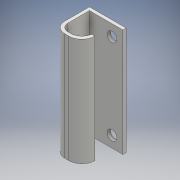
# Autodesk Inventor part: TopHook
Saved by Autodesk Inventor 2016 (Build 200138000, 138)
## iProperties
Created: 2015-06-09
Part Number: TopHook
Material: Generic
Document SubType Name: Modeling
Designer: Erin
Density: 1 g/cm^3
Appearance: Default
Author: Erin
Autodesk Inventor part; units mm, degrees
ref_plane "YZ Plane" through (0, 0, 0) normal (1, 0, 0) x (0, 1, 0)
ref_plane "XZ Plane" through (0, 0, 0) normal (0, 1, 0) x (-1, 0, 0)
ref_plane "XY Plane" through (0, 0, 0) normal (0, 0, 1) x (1, 0, 0)
sketch "Sketch1" plane through (0, 0, 0) normal (0, 0, 1) x (1, 0, 0)
  line L0 (-3.7865, -1.449) -> (13.2135, -1.449)
  line L1 (13.2135, -1.449) -> (13.2135, -2.949)
  line L2 (13.2135, -2.949) -> (-3.7865, -2.949)
  line L3 (-3.7865, -2.949) -> (-3.7865, -1.449)
  line L4 (-3.7865, -2.949) -> (-2.2865, -2.949)
  line L5 (-3.7865, -12.949) -> (-3.7865, -2.949)
  line L6 (3.2135, -16.449) -> (3.2135, -17.949)
  line L7 (3.2135, -17.949) -> (1.2135, -17.949)
  arc A0 (3.2135, -16.449) -> (7.7135, -11.949) centre (2.4495, -11.1849) ccw
  line L8 (7.7135, -11.949) -> (9.2135, -11.949)
  arc A1 (3.2135, -17.949) -> (9.2135, -11.949) centre (3.2135, -11.949) ccw
  arc A2 (-3.7865, -12.949) -> (1.2135, -17.949) centre (1.2135, -12.949) ccw
  arc A3 (-2.2865, -12.949) -> (1.2135, -16.449) centre (1.2135, -12.949) ccw
  line L9 (-3.7865, -12.949) -> (-2.2865, -12.949)
  line L10 (1.2135, -17.949) -> (1.2135, -16.449)
  line L11 (1.2135, -16.449) -> (3.2135, -16.449)
  line L12 (-2.2865, -2.949) -> (-2.2865, -12.949)
  point P0 (0, 0)
  dimension "d0" = 1.5
  dimension "d2" = 1.5
  dimension "d3" = 6
  dimension "d4" = 5
  dimension "d5" = 5
  dimension "d7" = 6
  dimension "d8" = 2
  dimension "d12" = 15.5
  dimension "d13" = 10
  dimension "d23" = 1.5
  constraints: 26 end point, 10 point on circle, 5 horizontal, 4 centre point, 4 parallel, 3 perpendicular, 2 point on line, 2 tangent, 1 vertical
  measures "d0" distance of L0.end L1.end
  measures "d2" distance of L8.start L8.end
  measures "d3" distance between parallel lines of L8 L7
  measures "d4" distance between parallel lines of L7 L9
  measures "d5" distance between parallel lines of L5 L10
  measures "d7" distance from line of L8.end L6
  measures "d8" distance of L6.end L7.end
  measures "d12" distance between parallel lines of L1 L12
  measures "d13" distance of L5.start L2.end
  measures "d23" distance between parallel lines of L12 L5
extrude "Extrusion1" add sketch "Sketch1" along normal blind 50
sketch "Sketch2" plane through (-2.2865, -2.949, 0) normal (0, -1, 0) x (1, 0, 0)
  line L0 (15.5, 50) -> (-1.5, 50) projected
  line L1 (10.5, 50) -> (10.5, 0) construction
  line L2 (15.5, 0) -> (-1.5, 0) projected
  line L3 (15.5, 0) -> (-1.5, 0) projected
  line L4 (-1.5, 0) -> (-1.5, 50) projected
  line L5 (15.5, 50) -> (-1.5, 50) projected
  line L6 (15.5, 0) -> (15.5, 50) projected
  circle A0 centre (10.5, 44.75) radius 2.25
  circle A1 centre (10.5, 5.25) radius 2.25
  point P0 (2.2865, 0)
  dimension "d14" = 5
  dimension "d15" = 4.5
  dimension "d16" = 4.5
  dimension "d18" = 3
  dimension "d19" = 3
  constraints: 4 point on line, 2 centre point, 2 end point, 1 vertical
  measures "d14" distance between parallel lines of L1 L6
  measures "d15" diameter of A0
  measures "d16" diameter of A1
  measures "d18" distance edge to line of A1 L2
  measures "d19" distance edge to line of A0 L0
extrude "Extrusion2" cut sketch "Sketch2" against normal blind 3 contours A0 | A1
body "Solid1"
